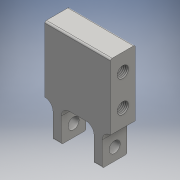
# Autodesk Inventor part: Profile_Middle_05
Saved by Autodesk Inventor 2016 (Build 200138000, 138)
## iProperties
Created: 2016-02-09
Part Number: Profile_Middle_05
Material: Generic
Document SubType Name: Modeling
Designer: nils
Density: 1 g/cm^3
Appearance: Default
Mass: 191.488 g
Surface Area: 349.032 cm^2
Volume: 191.488 cm^3
Author: nils
Autodesk Inventor part; units mm, degrees
ref_plane "YZ Plane" through (0, 0, 0) normal (1, 0, 0) x (0, 1, 0)
ref_plane "XZ Plane" through (0, 0, 0) normal (0, 1, 0) x (-1, 0, 0)
sketch "Sketch1" plane through (0, 0, 0) normal (1, 0, 0) x (0, 1, 0)
  line L0 (-15, 40) -> (15, 40)
  line L1 (15, 40) -> (15, -40)
  line L2 (15, -40) -> (-15, -40)
  line L3 (-15, -40) -> (-15, 40)
  line L4 (-15, 40) -> (15, -40) construction
  line L5 (15, 40) -> (-15, -40) construction
  point P0 (0, 0)
  dimension "d0" = 30
  dimension "d1" = 80
  constraints: 12 end point, 2 midpoint, 2 parallel, 1 horizontal, 1 perpendicular
  measures "d0" distance of L1.end L2.end
  measures "d1" distance of L0.end L1.end
extrude "Extrusion1" add sketch "Sketch1" along normal blind 80
sketch "Sketch2" plane through (80, 0, 0) normal (1, 0, 0) x (0, 0, -1)
  line L0 (-40, 15) -> (-40, -15) projected
  line L1 (-40, 0) -> (40, 0)
  line L2 (40, -15) -> (40, 15) projected
  line L3 (40, 15) -> (-40, 15) projected
  line L4 (0, 15) -> (0, -15)
  line L5 (-40, -15) -> (40, -15) projected
  point P0 (0, 0)
  point P1 (-19, 0)
  point P2 (19, 0)
  dimension "d4" = 19
  constraints: 4 end point, 4 midpoint, 2 point on line, 1 symmetric about line
  measures "d4" distance from line of L4 point (-19, 0)
hole "Hole1" at (80, 0, 19) at (80, 0, -19) direction (-1, 0, 0) diameter 13.835 depth 40 tip angle 118 thread size "M16x2" class "6H" standard "ISO Metric profile"
ref_plane "Work Plane1" through (40, 0, 0) normal (1, 0, 0) x (0, 0, -1)
mirror "Mirror1" about plane through (40, 0, 0) normal (1, 0, 0) of "Hole1"
sketch "Sketch9" plane through (0, -15, -40) normal (0, 0, -1) x (-1, 0, 0)
  line L0 (0, 0) -> (-80, 0) projected
  line L1 (0, 30) -> (-80, 30) projected
  line L2 (-80, 0) -> (-80, 30) projected
  line L3 (-20, 30) -> (-10, 30)
  line L4 (-10, 30) -> (-10, 0)
  line L5 (-10, 0) -> (-20, 0)
  line L6 (-20, 0) -> (-20, 30)
  line L7 (0, 30) -> (0, 0) projected
  line L8 (-60, 30) -> (-70, 30)
  line L9 (-70, 30) -> (-70, 0)
  line L10 (-70, 0) -> (-60, 0)
  line L11 (-60, 0) -> (-60, 30)
  dimension "d78" = 10
  dimension "d79" = 10
  dimension "d80" = 10
  dimension "d81" = 10
  constraints: 16 end point, 4 parallel, 4 point on line, 2 horizontal, 2 perpendicular
  measures "d78" distance between parallel lines of L6 L4
  measures "d79" distance between parallel lines of L4 L7
  measures "d80" distance between parallel lines of L2 L9
  measures "d81" distance between parallel lines of L9 L11
extrude "Extrusion4" add sketch "Sketch9" along normal blind 40 contours L0 L6 L1 L4 | L0 L9 L1 L11
hole "Hole6" at (70, 0, -65) direction (-1, 0, 0) diameter 13.5 end through all
fillet "Fillet12" radius 10 4 edges at (70, 0, -40) (60, 0, -40) (20, 0, -40) (10, 0, -40)
fillet "Fillet14" radius 2 4 edges at (15, 15, -80) (15, -15, -80) (65, 15, -80) (65, -15, -80)
fillet "Fillet15" radius 2 2 edges at (40, 15, 40) (40, -15, 40)
body "Solid1"
